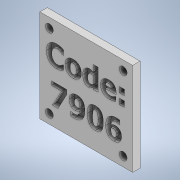
# Autodesk Inventor part: fireBoxSign
Saved by Autodesk Inventor 2021.2 (Build 252289000, 289)
## iProperties
Created: 2021-03-22
Part Number: fireBoxSign
Material: Generic
Document SubType Name: Modeling
Designer: robst
Density: 1 g/cm^3
Appearance: Default
Author: robst
Autodesk Inventor part; units mm, degrees
ref_plane "YZ Plane" through (0, 0, 0) normal (1, 0, 0) x (0, 1, 0)
ref_plane "XZ Plane" through (0, 0, 0) normal (0, 1, 0) x (-1, 0, 0)
ref_plane "XY Plane" through (0, 0, 0) normal (0, 0, 1) x (1, 0, 0)
sketch "Sketch2" plane through (0, 0, 0) normal (0, 0, 1) x (1, 0, 0)
  line L0 (-39.8907, -39.8907) -> (39.8907, -39.8907)
  line L1 (39.8907, -39.8907) -> (39.8907, 39.8907)
  line L2 (39.8907, 39.8907) -> (-39.8907, 39.8907)
  line L3 (-39.8907, 39.8907) -> (-39.8907, -39.8907)
  line L4 (-39.8907, -39.8907) -> (39.8907, 39.8907) construction
  line L5 (39.8907, -39.8907) -> (-39.8907, 39.8907) construction
  point P0 (0, 0)
  dimension "d6" = 79.7814
  dimension "d7" = 79.7814
  constraints: 12 end point, 2 midpoint, 2 parallel, 1 horizontal, 1 perpendicular
  measures "d6" distance of L1.end L2.end
  measures "d7" distance of L0.end L1.end
extrude "Extrusion2" add sketch "Sketch2" against normal blind 6.35
sketch "Sketch3" plane through (0, 0, 0) normal (0, 0, 1) x (1, 0, 0)
  line L0 (-31.75, -31.75) -> (31.75, -31.75) construction
  line L1 (31.75, -31.75) -> (31.75, 31.75) construction
  line L2 (31.75, 31.75) -> (-31.75, 31.75) construction
  line L3 (-31.75, 31.75) -> (-31.75, -31.75) construction
  line L4 (-31.75, -31.75) -> (31.75, 31.75) construction
  line L5 (31.75, -31.75) -> (-31.75, 31.75) construction
  point P0 (0, 0)
  dimension "d10" = 63.5
  dimension "d11" = 63.5
  constraints: 12 end point, 4 coincident, 2 midpoint, 2 parallel, 1 horizontal, 1 perpendicular
  measures "d10" distance of L1.end L2.end
  measures "d11" distance of L0.end L1.end
hole "Hole1" at (-31.75, 31.75, 0) at (31.75, 31.75, 0) at (31.75, -31.75, 0) at (-31.75, -31.75, 0) direction (0, 0, -1) diameter 6.7564 end through all clearance for "Socket Head Cap Screw" size "1/4" standard "Ansi Unified Screw Threads"
sketch "Sketch4" plane through (0, 0, 0) normal (0, 0, 1) x (1, 0, 0)
  line L0 (-28.575, -28.575) -> (28.575, -28.575) construction
  line L1 (28.575, -28.575) -> (28.575, 28.575) construction
  line L2 (28.575, 28.575) -> (-28.575, 28.575) construction
  line L3 (-28.575, 28.575) -> (-28.575, -28.575) construction
  line L4 (-28.575, -28.575) -> (28.575, 28.575) construction
  line L5 (28.575, -28.575) -> (-28.575, 28.575) construction
  line L6 (-28.575, 0) -> (28.575, 0) construction
  spline S0 degree 2 poles (-25.5894, 4.7342) (-29.5949, 4.7342) (-34.2921, 9.5754) (-34.2921, 13.9556) knots 0 0 0 1 2 2 2
  spline S1 degree 2 poles (-34.2921, 13.9556) (-34.2921, 18.1773) (-29.5805, 23.2058) (-25.575, 23.2058) knots 0 0 0 1 2 2 2
  spline S2 degree 2 poles (-25.575, 23.2058) (-24.5231, 23.2058) (-22.8229, 22.9609) (-22.0449, 22.7591) knots 0 0 0 1 2 2 2
  spline S3 degree 2 poles (-22.0449, 22.7591) (-21.4397, 22.5718) (-20.0133, 21.9523) (-19.5666, 21.7217) knots 0 0 0 1 2 2 2
  line L7 (-19.5666, 21.7217) -> (-19.5666, 17.4857)
  line L8 (-19.5666, 17.4857) -> (-20.0133, 17.4857)
  spline S4 degree 2 poles (-20.0133, 17.4857) (-20.3447, 17.7738) (-21.3245, 18.5807) (-21.944, 18.9553) knots 0 0 0 1 2 2 2
  spline S5 degree 2 poles (-21.944, 18.9553) (-22.5636, 19.3443) (-24.0477, 19.8775) (-24.8689, 19.8775) knots 0 0 0 1 2 2 2
  spline S6 degree 2 poles (-24.8689, 19.8775) (-25.8343, 19.8775) (-27.4336, 19.2723) (-28.1685, 18.5087) knots 0 0 0 1 2 2 2
  spline S7 degree 2 poles (-28.1685, 18.5087) (-28.8313, 17.8315) (-29.6814, 15.5117) (-29.6814, 13.9412) knots 0 0 0 1 2 2 2
  spline S8 degree 2 poles (-29.6814, 13.9412) (-29.6814, 12.2842) (-28.8024, 10.0221) (-28.082, 9.3305) knots 0 0 0 1 2 2 2
  spline S9 degree 2 poles (-28.082, 9.3305) (-27.3904, 8.6533) (-25.6902, 8.0625) (-24.8401, 8.0625) knots 0 0 0 1 2 2 2
  spline S10 degree 2 poles (-24.8401, 8.0625) (-23.9612, 8.0625) (-22.3619, 8.6533) (-21.8144, 9.0135) knots 0 0 0 1 2 2 2
  spline S11 degree 2 poles (-21.8144, 9.0135) (-21.2092, 9.3737) (-20.3015, 10.1374) (-19.9701, 10.4399) knots 0 0 0 1 2 2 2
  line L9 (-19.9701, 10.4399) -> (-19.5666, 10.4399)
  line L10 (-19.5666, 10.4399) -> (-19.5666, 6.2615)
  spline S12 degree 2 poles (-19.5666, 6.2615) (-20.0565, 6.031) (-21.3389, 5.4546) (-22.0305, 5.2529) knots 0 0 0 1 2 2 2
  spline S13 degree 2 poles (-22.0305, 5.2529) (-22.8662, 4.9935) (-24.3214, 4.7342) (-25.5894, 4.7342) knots 0 0 0 1 2 2 2
  spline S14 degree 2 poles (-4.3081, 11.7799) (-4.3081, 8.466) (-7.9246, 4.6622) (-11.2242, 4.6622) knots 0 0 0 1 2 2 2
  spline S15 degree 2 poles (-11.2242, 4.6622) (-14.5093, 4.6622) (-18.1546, 8.466) (-18.1546, 11.7799) knots 0 0 0 1 2 2 2
  spline S16 degree 2 poles (-18.1546, 11.7799) (-18.1546, 15.1227) (-14.5093, 18.9121) (-11.2242, 18.9121) knots 0 0 0 1 2 2 2
  spline S17 degree 2 poles (-11.2242, 18.9121) (-7.939, 18.9121) (-4.3081, 15.1083) (-4.3081, 11.7799) knots 0 0 0 1 2 2 2
  spline S18 degree 2 poles (-8.5874, 11.7511) (-8.5874, 12.947) (-8.9765, 14.5463) (-9.3223, 15.0218) knots 0 0 0 1 2 2 2
  spline S19 degree 2 poles (-9.3223, 15.0218) (-9.6969, 15.5261) (-10.6334, 15.9151) (-11.2242, 15.9151) knots 0 0 0 1 2 2 2
  spline S20 degree 2 poles (-11.2242, 15.9151) (-11.8005, 15.9151) (-12.7082, 15.5693) (-13.0829, 15.0794) knots 0 0 0 1 2 2 2
  spline S21 degree 2 poles (-13.0829, 15.0794) (-13.4431, 14.6184) (-13.8753, 12.9902) (-13.8753, 11.7511) knots 0 0 0 1 2 2 2
  spline S22 degree 2 poles (-13.8753, 11.7511) (-13.8753, 10.5264) (-13.4719, 9.0135) (-13.1405, 8.5524) knots 0 0 0 1 2 2 2
  spline S23 degree 2 poles (-13.1405, 8.5524) (-12.8091, 8.0914) (-11.8005, 7.6591) (-11.1953, 7.6591) knots 0 0 0 1 2 2 2
  spline S24 degree 2 poles (-11.1953, 7.6591) (-10.6911, 7.6591) (-9.6536, 8.0914) (-9.3367, 8.5236) knots 0 0 0 1 2 2 2
  spline S25 degree 2 poles (-9.3367, 8.5236) (-8.9765, 9.0279) (-8.5874, 10.4832) (-8.5874, 11.7511) knots 0 0 0 1 2 2 2
  line L11 (10.1003, 5.08) -> (5.9219, 5.08)
  line L12 (5.9219, 5.08) -> (5.9219, 6.4776)
  spline S26 degree 2 poles (5.9219, 6.4776) (5.5184, 6.1462) (4.481, 5.3826) (4.0776, 5.1809) knots 0 0 0 1 2 2 2
  spline S27 degree 2 poles (4.0776, 5.1809) (3.5877, 4.9503) (2.6079, 4.7054) (1.9307, 4.7054) knots 0 0 0 1 2 2 2
  spline S28 degree 2 poles (1.9307, 4.7054) (-0.3602, 4.7054) (-3.0402, 8.5092) (-3.0402, 11.6791) knots 0 0 0 1 2 2 2
  spline S29 degree 2 poles (-3.0402, 11.6791) (-3.0402, 13.4369) (-2.1324, 16.016) (-1.34, 16.967) knots 0 0 0 1 2 2 2
  spline S30 degree 2 poles (-1.34, 16.967) (-0.6052, 17.8459) (1.4697, 18.8545) (2.6223, 18.8545) knots 0 0 0 1 2 2 2
  spline S31 degree 2 poles (2.6223, 18.8545) (3.6741, 18.8545) (5.0285, 18.4078) (5.9219, 17.9467) knots 0 0 0 1 2 2 2
  line L13 (5.9219, 17.9467) -> (5.9219, 23.6525)
  line L14 (5.9219, 23.6525) -> (10.1003, 23.6525)
  line L15 (10.1003, 23.6525) -> (10.1003, 5.08)
  line L16 (5.9219, 8.7686) -> (5.9219, 15.3532)
  spline S32 degree 2 poles (5.9219, 15.3532) (5.6193, 15.5117) (4.6107, 15.7134) (4.2505, 15.7134) knots 0 0 0 1 2 2 2
  spline S33 degree 2 poles (4.2505, 15.7134) (2.752, 15.7134) (1.2391, 13.6098) (1.2391, 11.7223) knots 0 0 0 1 2 2 2
  spline S34 degree 2 poles (1.2391, 11.7223) (1.2391, 9.7339) (2.4494, 7.9617) (3.7894, 7.9617) knots 0 0 0 1 2 2 2
  spline S35 degree 2 poles (3.7894, 7.9617) (4.3369, 7.9617) (5.4608, 8.3939) (5.9219, 8.7686) knots 0 0 0 1 2 2 2
  spline S36 degree 2 poles (20.1718, 4.7198) (16.368, 4.7198) (12.3192, 8.3507) (12.3192, 11.7079) knots 0 0 0 1 2 2 2
  spline S37 degree 2 poles (12.3192, 11.7079) (12.3192, 14.993) (16.0942, 18.9121) (19.4946, 18.9121) knots 0 0 0 1 2 2 2
  spline S38 degree 2 poles (19.4946, 18.9121) (22.5636, 18.9121) (25.6758, 15.5837) (25.6758, 12.5003) knots 0 0 0 1 2 2 2
  line L17 (25.6758, 12.5003) -> (25.6758, 10.9875)
  line L18 (25.6758, 10.9875) -> (16.4976, 10.9875)
  spline S39 degree 2 poles (16.4976, 10.9875) (16.5553, 10.0509) (17.2325, 8.8118) (17.78, 8.4372) knots 0 0 0 1 2 2 2
  spline S40 degree 2 poles (17.78, 8.4372) (18.3131, 8.0625) (19.754, 7.7456) (20.6041, 7.7456) knots 0 0 0 1 2 2 2
  spline S41 degree 2 poles (20.6041, 7.7456) (21.3245, 7.7456) (22.7365, 8.0625) (23.3272, 8.3363) knots 0 0 0 1 2 2 2
  spline S42 degree 2 poles (23.3272, 8.3363) (23.8459, 8.5524) (24.7105, 9.0855) (24.9842, 9.2873) knots 0 0 0 1 2 2 2
  line L19 (24.9842, 9.2873) -> (25.4309, 9.2873)
  line L20 (25.4309, 9.2873) -> (25.4309, 5.8292)
  spline S43 degree 2 poles (25.4309, 5.8292) (24.9122, 5.6275) (24.0765, 5.2817) (23.3272, 5.1088) knots 0 0 0 1 2 2 2
  spline S44 degree 2 poles (23.3272, 5.1088) (22.65, 4.9215) (21.2092, 4.7198) (20.1718, 4.7198) knots 0 0 0 1 2 2 2
  spline S45 degree 2 poles (21.555, 13.5089) (21.5262, 14.8345) (20.3591, 16.2321) (19.1632, 16.2321) knots 0 0 0 1 2 2 2
  spline S46 degree 2 poles (19.1632, 16.2321) (17.9385, 16.2321) (16.5553, 14.7625) (16.4832, 13.5089) knots 0 0 0 1 2 2 2
  line L21 (16.4832, 13.5089) -> (21.555, 13.5089)
  line L22 (32.7792, 5.08) -> (28.5575, 5.08)
  line L23 (28.5575, 5.08) -> (28.5575, 9.7771)
  line L24 (28.5575, 9.7771) -> (32.7792, 9.7771)
  line L25 (32.7792, 9.7771) -> (32.7792, 5.08)
  line L26 (32.7792, 13.7971) -> (28.5575, 13.7971)
  line L27 (28.5575, 13.7971) -> (28.5575, 18.4942)
  line L28 (28.5575, 18.4942) -> (32.7792, 18.4942)
  line L29 (32.7792, 18.4942) -> (32.7792, 13.7971)
  line L30 (-16.6706, -10.0168) -> (-24.2638, -24.2668)
  line L31 (-24.2638, -24.2668) -> (-29.2203, -24.2668)
  line L32 (-29.2203, -24.2668) -> (-21.2812, -9.8439)
  line L33 (-21.2812, -9.8439) -> (-29.7534, -9.8439)
  line L34 (-29.7534, -9.8439) -> (-29.7534, -6.4868)
  line L35 (-29.7534, -6.4868) -> (-16.6706, -6.4868)
  line L36 (-16.6706, -6.4868) -> (-16.6706, -10.0168)
  spline S47 degree 2 poles (-1.1671, -14.3826) (-1.1671, -16.6447) (-2.2189, -20.4197) (-3.3283, -21.7741) knots 0 0 0 1 2 2 2
  spline S48 degree 2 poles (-3.3283, -21.7741) (-4.481, -23.1429) (-7.8814, -24.6126) (-10.3597, -24.6126) knots 0 0 0 1 2 2 2
  spline S49 degree 2 poles (-10.3597, -24.6126) (-11.1953, -24.6126) (-13.0108, -24.3964) (-13.3134, -24.31) knots 0 0 0 1 2 2 2
  line L37 (-13.3134, -24.31) -> (-13.3134, -20.8231)
  line L38 (-13.3134, -20.8231) -> (-12.9676, -20.8231)
  spline S50 degree 2 poles (-12.9676, -20.8231) (-12.6362, -20.996) (-11.3971, -21.3707) (-10.3164, -21.3707) knots 0 0 0 1 2 2 2
  spline S51 degree 2 poles (-10.3164, -21.3707) (-9.4375, -21.3707) (-7.8094, -20.9096) (-7.233, -20.4053) knots 0 0 0 1 2 2 2
  spline S52 degree 2 poles (-7.233, -20.4053) (-6.6135, -19.8722) (-5.8066, -18.3017) (-5.6625, -17.1202) knots 0 0 0 1 2 2 2
  spline S53 degree 2 poles (-5.6625, -17.1202) (-6.6135, -17.7109) (-8.256, -18.3449) (-9.4807, -18.3449) knots 0 0 0 1 2 2 2
  spline S54 degree 2 poles (-9.4807, -18.3449) (-10.3885, -18.3449) (-12.0743, -17.855) (-12.7659, -17.3363) knots 0 0 0 1 2 2 2
  spline S55 degree 2 poles (-12.7659, -17.3363) (-13.688, -16.6303) (-14.7686, -14.3682) (-14.7686, -12.5815) knots 0 0 0 1 2 2 2
  spline S56 degree 2 poles (-14.7686, -12.5815) (-14.7686, -11.1839) (-13.8177, -8.8353) (-12.9532, -7.9708) knots 0 0 0 1 2 2 2
  spline S57 degree 2 poles (-12.9532, -7.9708) (-12.0887, -7.1063) (-9.5816, -6.1265) (-8.0399, -6.1265) knots 0 0 0 1 2 2 2
  spline S58 degree 2 poles (-8.0399, -6.1265) (-6.4838, -6.1265) (-4.0776, -6.9911) (-3.2131, -7.8988) knots 0 0 0 1 2 2 2
  spline S59 degree 2 poles (-3.2131, -7.8988) (-2.2045, -8.9074) (-1.1671, -12.106) (-1.1671, -14.3826) knots 0 0 0 1 2 2 2
  spline S60 degree 2 poles (-5.5905, -13.7198) (-5.5905, -12.2645) (-6.0804, -10.3914) (-6.527, -9.8727) knots 0 0 0 1 2 2 2
  spline S61 degree 2 poles (-6.527, -9.8727) (-6.8296, -9.4837) (-7.6076, -9.1523) (-8.0543, -9.1523) knots 0 0 0 1 2 2 2
  spline S62 degree 2 poles (-8.0543, -9.1523) (-8.4577, -9.1523) (-9.207, -9.4693) (-9.5528, -9.8727) knots 0 0 0 1 2 2 2
  spline S63 degree 2 poles (-9.5528, -9.8727) (-9.8554, -10.2185) (-10.2876, -11.5585) (-10.2876, -12.351) knots 0 0 0 1 2 2 2
  spline S64 degree 2 poles (-10.2876, -12.351) (-10.2876, -13.2155) (-9.841, -14.3249) (-9.4663, -14.6563) knots 0 0 0 1 2 2 2
  spline S65 degree 2 poles (-9.4663, -14.6563) (-9.0773, -14.9877) (-8.1119, -15.2471) (-7.5068, -15.2471) knots 0 0 0 1 2 2 2
  spline S66 degree 2 poles (-7.5068, -15.2471) (-7.0025, -15.2471) (-5.9507, -14.9733) (-5.6193, -14.8292) knots 0 0 0 1 2 2 2
  spline S67 degree 2 poles (-5.6193, -14.8292) (-5.6193, -14.6996) (-5.5905, -14.2097) (-5.5905, -13.7198) knots 0 0 0 1 2 2 2
  spline S68 degree 2 poles (14.639, -15.3768) (14.639, -17.6821) (13.9041, -21.1401) (13.0829, -22.3072) knots 0 0 0 1 2 2 2
  spline S69 degree 2 poles (13.0829, -22.3072) (12.276, -23.4599) (9.6681, -24.6414) (7.795, -24.6414) knots 0 0 0 1 2 2 2
  spline S70 degree 2 poles (7.795, -24.6414) (5.9075, -24.6414) (3.3139, -23.4599) (2.4927, -22.2784) knots 0 0 0 1 2 2 2
  spline S71 degree 2 poles (2.4927, -22.2784) (1.6714, -21.1113) (0.9365, -17.6821) (0.9365, -15.3768) knots 0 0 0 1 2 2 2
  spline S72 degree 2 poles (0.9365, -15.3768) (0.9365, -13.0138) (1.6714, -9.671) (2.5071, -8.4607) knots 0 0 0 1 2 2 2
  spline S73 degree 2 poles (2.5071, -8.4607) (3.3428, -7.2792) (5.9795, -6.1265) (7.795, -6.1265) knots 0 0 0 1 2 2 2
  spline S74 degree 2 poles (7.795, -6.1265) (9.7113, -6.1265) (12.276, -7.3369) (13.0973, -8.5328) knots 0 0 0 1 2 2 2
  spline S75 degree 2 poles (13.0973, -8.5328) (13.9041, -9.6998) (14.639, -13.1435) (14.639, -15.3768) knots 0 0 0 1 2 2 2
  spline S76 degree 2 poles (10.1579, -15.3768) (10.1579, -12.0772) (9.0773, -9.4117) (7.795, -9.4117) knots 0 0 0 1 2 2 2
  spline S77 degree 2 poles (7.795, -9.4117) (6.5126, -9.4117) (5.4176, -12.0772) (5.4176, -15.3912) knots 0 0 0 1 2 2 2
  spline S78 degree 2 poles (5.4176, -15.3912) (5.4176, -18.6475) (6.5126, -21.3563) (7.795, -21.3563) knots 0 0 0 1 2 2 2
  spline S79 degree 2 poles (7.795, -21.3563) (9.0629, -21.3563) (10.1579, -18.6475) (10.1579, -15.3768) knots 0 0 0 1 2 2 2
  spline S80 degree 2 poles (30.3441, -18.2152) (30.3441, -21.0249) (26.7853, -24.6414) (23.673, -24.6414) knots 0 0 0 1 2 2 2
  spline S81 degree 2 poles (23.673, -24.6414) (22.1169, -24.6414) (19.6819, -23.7481) (18.8318, -22.8691) knots 0 0 0 1 2 2 2
  spline S82 degree 2 poles (18.8318, -22.8691) (17.8232, -21.8461) (16.7426, -18.6042) (16.7426, -16.3421) knots 0 0 0 1 2 2 2
  spline S83 degree 2 poles (16.7426, -16.3421) (16.7426, -14.008) (17.7512, -10.377) (18.8894, -8.9794) knots 0 0 0 1 2 2 2
  spline S84 degree 2 poles (18.8894, -8.9794) (19.9701, -7.6538) (23.4857, -6.1554) (25.8919, -6.1554) knots 0 0 0 1 2 2 2
  spline S85 degree 2 poles (25.8919, -6.1554) (26.7709, -6.1554) (28.5287, -6.3859) (28.8457, -6.4579) knots 0 0 0 1 2 2 2
  line L39 (28.8457, -6.4579) -> (28.8457, -9.9448)
  line L40 (28.8457, -9.9448) -> (28.5287, -9.9448)
  spline S86 degree 2 poles (28.5287, -9.9448) (28.2117, -9.7863) (26.7709, -9.3973) (25.8487, -9.3973) knots 0 0 0 1 2 2 2
  spline S87 degree 2 poles (25.8487, -9.3973) (23.7595, -9.3973) (21.483, -11.6018) (21.2092, -13.6477) knots 0 0 0 1 2 2 2
  spline S88 degree 2 poles (21.2092, -13.6477) (22.0881, -13.0858) (23.8892, -12.423) (25.0274, -12.423) knots 0 0 0 1 2 2 2
  spline S89 degree 2 poles (25.0274, -12.423) (25.9928, -12.423) (27.6786, -12.9417) (28.327, -13.4316) knots 0 0 0 1 2 2 2
  spline S90 degree 2 poles (28.327, -13.4316) (29.2491, -14.1376) (30.3441, -16.4286) (30.3441, -18.2152) knots 0 0 0 1 2 2 2
  spline S91 degree 2 poles (25.1427, -20.8952) (25.4885, -20.4629) (25.8631, -19.4543) (25.8631, -18.4313) knots 0 0 0 1 2 2 2
  spline S92 degree 2 poles (25.8631, -18.4313) (25.8631, -17.5668) (25.4309, -16.443) (25.0418, -16.1116) knots 0 0 0 1 2 2 2
  spline S93 degree 2 poles (25.0418, -16.1116) (24.6384, -15.7658) (23.6442, -15.5208) (23.0823, -15.5208) knots 0 0 0 1 2 2 2
  spline S94 degree 2 poles (23.0823, -15.5208) (22.6068, -15.5208) (21.627, -15.7658) (21.1948, -15.9387) knots 0 0 0 1 2 2 2
  spline S95 degree 2 poles (21.1948, -15.9387) (21.1948, -16.054) (21.166, -16.6015) (21.166, -17.0193) knots 0 0 0 1 2 2 2
  spline S96 degree 2 poles (21.166, -17.0193) (21.166, -18.561) (21.6991, -20.4197) (22.1169, -20.8952) knots 0 0 0 1 2 2 2
  spline S97 degree 2 poles (22.1169, -20.8952) (22.4195, -21.2842) (23.2264, -21.6156) (23.6586, -21.6156) knots 0 0 0 1 2 2 2
  spline S98 degree 2 poles (23.6586, -21.6156) (24.0188, -21.6156) (24.8545, -21.2554) (25.1427, -20.8952) knots 0 0 0 1 2 2 2
  point P0 (0, 0)
  dimension "d19" = 57.15
  dimension "d20" = 57.15
  constraints: 14 end point, 4 midpoint, 2 horizontal, 2 parallel, 1 perpendicular
  measures "d19" distance of L1.end L2.end
  measures "d20" distance of L0.end L1.end
extrude "Extrusion3" cut sketch "Sketch4" against normal blind 4.2333
equation "\"d6\" = outerWidth"
equation "\"d7\" = outerHeight"
equation "\"d8\" = thickness"
equation "\"d10\" = centerWidthBoltHole"
equation "\"d11\" = centerHeightBoltHole"
equation "\"d19\" = textBoxWidth"
equation "\"d20\" = textBoxHeight"
equation "\"d21\" = textDepth"
equation "\"centerWidthBoltHole\" = 63.5"
equation "\"centerHeightBoltHole\" = 63.5"
equation "\"boltHoleClearance\" = 6.7564"
equation "\"thickness\" = 6.35"
equation "\"textHeight\" = 12.7"
equation "\"textDepth\" = 0.666667 * thickness"
equation "\"outerWidth\" = 79.7814"
equation "\"outerHeight\" = 79.7814"
equation "\"textBoxWidth\" = 57.15"
equation "\"textBoxHeight\" = 57.15"
body "Solid2"
